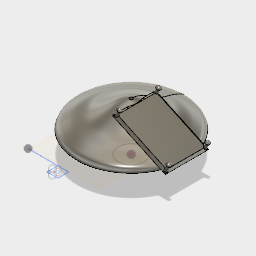
modiTOP v4 (Autodesk Fusion 360 design; units mm, degrees)
Autodesk Fusion 360 part; units mm, degrees
note: some values were not read from the file. Set by a fixed rule: which sketch regions a step uses.
sketch "Sketch1" plane through (0, 0, 0) normal (0, 1, 0) x (1, 0, 0)
  line L0 (-40.284, 39.4847) -> (20.716, 39.4847)
  line L1 (20.716, 39.4847) -> (20.716, -51.0153)
  line L2 (20.716, -51.0153) -> (-40.284, -51.0153)
  line L3 (-40.284, -51.0153) -> (-40.284, 39.4847)
  dimension "d1" = 61
  dimension "d2" = 90.5
  measures "d1" distance of L0.start L0.end
  measures "d2" distance of L0.start L2.end
extrude "Extrude1" add sketch "Sketch1" along normal blind 10 makes body 1
shell "Shell1" thickness 2 outward yes removed faces 1 at (-19.9507, 10, -9.3181) on bodies 1
sketch "Sketch2" plane through (0, 0, 0) normal (0, 1, 0) x (-1, 0, 0)
  line L0 (40.284, 51.0153) -> (-20.716, 51.0153)
  line L1 (-20.716, 51.0153) -> (-20.716, -39.4847)
  line L2 (-20.716, -39.4847) -> (40.284, -39.4847)
  line L3 (40.284, -39.4847) -> (40.284, 51.0153)
  line L4 (40.284, 51.0153) -> (9.784, 51.0153)
  line L5 (9.784, 51.0153) -> (9.784, 5.7653)
  circle A0 centre (9.784, 5.7653) radius 9
  dimension "d6" = 45.25
  dimension "d7" = 18
  measures "d6" distance of L4.end L5.end
  measures "d7" diameter of A0
extrude "Extrude2" cut sketch "Sketch2" against normal blind 3 contours A0 bodies 1
sketch "Sketch3" plane through (0, 10, 0) normal (0, 1, 0) x (-1, 0, 0)
  line L0 (40.284, 51.0153) -> (40.284, -39.4847)
  line L1 (40.284, -39.4847) -> (-20.716, -39.4847)
  line L2 (-20.716, -39.4847) -> (-20.716, 51.0153)
  line L3 (-20.716, 51.0153) -> (40.284, 51.0153)
  line L4 (42.284, 53.0153) -> (-22.716, 53.0153)
  line L5 (-22.716, 53.0153) -> (-22.716, -41.4847)
  line L6 (-22.716, -41.4847) -> (42.284, -41.4847)
  line L7 (42.284, -41.4847) -> (42.284, 53.0153)
  line L8 (42.284, -41.4847) -> (14.784, -41.4847)
  line L9 (14.784, -41.4847) -> (4.784, -41.4847)
  line L10 (4.784, -41.4847) -> (-22.716, -41.4847)
  line L11 (14.784, -41.4847) -> (4.784, -41.4847)
  line L12 (4.784, -41.4847) -> (4.784, -51.4847)
  line L13 (4.784, -51.4847) -> (14.784, -51.4847)
  line L14 (14.784, -51.4847) -> (14.784, -41.4847)
  line L15 (4.784, -51.4847) -> (9.784, -51.4847)
  line L16 (9.784, -51.4847) -> (9.784, -46.4847)
  circle A0 centre (9.784, -46.4847) radius 1.5
  dimension "d10" = 27.5
  dimension "d11" = 10
  dimension "d12" = 27.5
  dimension "d13" = 10
  dimension "d14" = 10
  dimension "d15" = 5
  dimension "d16" = 5
  dimension "d17" = 3
  measures "d10" distance of L6.end L8.end
  measures "d11" distance of L8.end L9.end
  measures "d12" distance of L9.end L5.end
  measures "d13" distance of L8.end L9.end
  measures "d14" distance of L8.end L13.end
  measures "d15" distance of L12.end L15.end
  measures "d16" distance of L15.end L16.end
  measures "d17" diameter of A0
extrude "Extrude3" add sketch "Sketch3" against normal blind 5 contours L6 L9 L11 L12 L13 L14 L15 bodies 1
sketch "Sketch4" plane through (0, 10, 0) normal (0, 1, 0) x (-1, 0, 0)
  circle A0 centre (9.784, -46.4847) radius 1.5
  line L0 (40.284, 51.0153) -> (40.284, -39.4847)
  line L1 (40.284, -39.4847) -> (-20.716, -39.4847)
  line L2 (-20.716, -39.4847) -> (-20.716, 51.0153)
  line L3 (-20.716, 51.0153) -> (40.284, 51.0153)
  line L4 (42.284, 53.0153) -> (-22.716, 53.0153)
  line L5 (-22.716, 53.0153) -> (-22.716, -41.4847)
  line L6 (-22.716, -41.4847) -> (4.784, -41.4847)
  line L7 (4.784, -41.4847) -> (4.784, -51.4847)
  line L8 (4.784, -51.4847) -> (14.784, -51.4847)
  line L9 (14.784, -51.4847) -> (14.784, -41.4847)
  line L10 (14.784, -41.4847) -> (42.284, -41.4847)
  line L11 (42.284, -41.4847) -> (42.284, 53.0153)
  line L12 (42.284, 53.0153) -> (14.784, 53.0153)
  line L13 (14.784, 53.0153) -> (4.784, 53.0153)
  line L14 (4.784, 53.0153) -> (4.784, 63.0153)
  line L15 (4.784, 63.0153) -> (14.784, 63.0153)
  line L16 (14.784, 63.0153) -> (14.784, 53.0153)
  line L17 (14.784, 63.0153) -> (9.784, 63.0153)
  line L18 (14.784, 58.0153) -> (14.784, 63.0153)
  circle A1 centre (9.784, 58.0153) radius 1.5
  dimension "d20" = 27.5
  dimension "d21" = 10
  dimension "d22" = 10
  dimension "d23" = 5
  dimension "d24" = 5
  dimension "d25" = 3
  measures "d20" distance of L4.start L12.end
  measures "d21" distance of L12.end L13.end
  measures "d22" distance of L12.end L15.end
  measures "d23" distance of L15.end L17.end
  measures "d24" distance of L15.end L18.start
  measures "d25" diameter of A1
extrude "Extrude4" add sketch "Sketch4" against normal blind 5 contours L4 L13 L14 L15 L16 L17 L18 bodies 1
sketch "Sketch5" plane through (0, 0, 0) normal (0, 1, 0) x (1, 0, 0)
  circle A0 centre (0, 0) radius 12
  dimension "d28" = 24
  measures "d28" diameter of A0
extrude "Extrude5" add sketch "Sketch5" along normal blind 10 separate body makes body 2
extrude "Extrude6" add 1 faces at (1.8223, 10, -1.3289) along direction (0, 1, 0) blind 10 on bodies 2 bodies 2
shell "Shell2" thickness 2 removed faces 1 at (1.8223, 20, -1.3289) on bodies 2
sketch "Sketch6" plane through (0, 0, 0) normal (1, 0, 0) x (0, 0, -1)
  line L0 (-10, 20) -> (10, 20)
  line L1 (0, 20) -> (0, 45)
  line L2 (0, 20) -> (50, 20)
  spline S0 degree 5 poles (0, 45) (0.3016, 44.9569) (0.8982, 44.8674) (1.7738, 44.7229) (2.9022, 44.5101) (4.2485, 44.21) (5.5325, 43.8749) (6.7585, 43.5032) (7.9341, 43.0921) (9.0709, 42.6377) (10.1838, 42.1352) (11.2892, 41.5803) (12.4029, 40.9706) (13.5381, 40.3065) (14.7037, 39.5927) (15.9035, 38.8381) (17.137, 38.054) (18.3994, 37.2538) (19.6817, 36.4513) (20.9713, 35.6603) (22.2522, 34.8928) (23.5079, 34.1595) (24.7246, 33.4693) (25.8944, 32.8291) (27.018, 32.2438) (28.1088, 31.7161) (29.1922, 31.246) (30.2969, 30.8301) (31.4488, 30.4613) (32.6642, 30.128) (33.941, 29.8131) (35.2609, 29.4959) (36.5968, 29.1563) (37.9194, 28.7782) (39.2032, 28.3529) (40.4343, 27.8835) (41.6132, 27.3855) (42.7472, 26.8789) (43.8449, 26.3817) (44.9104, 25.9032) (45.9361, 25.4363) (46.9006, 24.9552) (47.7763, 24.425) (48.5341, 23.8086) (49.1499, 23.0753) (49.61, 22.207) (49.8482, 21.3973) (49.9528, 20.7243) (49.9897, 20.2463) (50, 20) knots 0 0 0 0 0 0 0.022222 0.044444 0.066667 0.088889 0.111111 0.133333 0.155556 0.177778 0.2 0.222222 0.244444 0.266667 0.288889 0.311111 0.333333 0.355556 0.377778 0.4 0.422222 0.444444 0.466667 0.488889 0.511111 0.533333 0.555556 0.577778 0.6 0.622222 0.644444 0.666667 0.688889 0.711111 0.733333 0.755556 0.777778 0.8 0.822222 0.844444 0.866667 0.888889 0.911111 0.933333 0.955556 0.977778 1 1 1 1 1 1
  point P0 (7.2369, 43.3286)
  point P1 (12.8037, 40.7307)
  point P2 (19.6695, 36.4628)
  point P3 (26.5353, 32.5)
  point P4 (31.9166, 30.3393)
  point P5 (38.7823, 28.4837)
  point P6 (44.5348, 26.0714)
  point P7 (48.4315, 23.8446)
  dimension "d34" = 25
  dimension "d35" = 50
  measures "d34" distance of L1.start L1.end
  measures "d35" distance of L1.start L2.end
revolve "Revolve1" add sketch "Sketch6" angle 360 about axis through (0, 1.75, 0) along (0, 1, 0) bodies 2
sketch "Sketch7" plane through (0, 0, 0) normal (0, -1, 0) x (1, 0, 0)
  circle A0 centre (0, 0) radius 12
  circle A1 centre (0, 0) radius 11
  dimension "d37" = 22
  measures "d37" diameter of A1
extrude "Extrude7" cut sketch "Sketch7" against normal blind 10 contours A1 bodies 2
sketch "Sketch8" plane through (0, 20, 0) normal (0, -1, 0) x (1, 0, 0)
  circle A0 centre (0, 0) radius 10
  circle A1 centre (0, 0) radius 12
  line L0 (0, 0) -> (-6, -10.3923)
  line L1 (0, 0) -> (12, 0) construction
  line L2 (0, 0) -> (6, -10.3923)
  line L3 (0, 0) -> (12, 0) construction
  line L4 (6, -10.3923) -> (6, -13.3923)
  line L5 (6, -13.3923) -> (-6, -13.3923)
  line L6 (-6, -13.3923) -> (-6, -10.3923)
  line L7 (0, 0) -> (-6, 10.3923)
  line L8 (0, 0) -> (12, 0) construction
  line L9 (0, 0) -> (6, 10.3923)
  line L10 (0, 0) -> (12, 0) construction
  line L11 (6, 10.3923) -> (6, 13.3923)
  line L12 (6, 13.3923) -> (-6, 13.3923)
  line L13 (-6, 13.3923) -> (-6, 10.3923)
  dimension "d40" = 24
  dimension "d42" = 120
  dimension "d43" = 60
  dimension "d45" = 3
  dimension "d46" = 120
  dimension "d47" = 60
  dimension "d48" = 3
  measures "d40" diameter of A1
  measures "d42" angle of L0 L1
  measures "d43" angle of L2 L3
  measures "d45" distance of L0.end L5.end
  measures "d46" angle of L7 L8
  measures "d47" angle of L9 L10
  measures "d48" distance of L7.end L12.end
extrude "Extrude8" add sketch "Sketch8" along normal blind 20 contours A1 L11 L12 L13 | A1 L4 L5 L6 bodies 2
sketch "Sketch9" plane through (0, 0, -13.3923) normal (0, 0, -1) x (-1, 0, 0)
  line L0 (6, 20) -> (-6, 20)
  line L1 (-6, 20) -> (-6, 0)
  line L2 (-6, 0) -> (6, 0)
  line L3 (6, 0) -> (6, 20)
  line L4 (6, 0) -> (0, 0)
  line L5 (0, 0) -> (0, 5)
  circle A0 centre (0, 5) radius 1.5
  dimension "d51" = 5
  dimension "d52" = 3
  measures "d51" distance of L4.end L5.end
  measures "d52" diameter of A0
extrude "Extrude9" cut sketch "Sketch9" against normal blind 100 contours A0 bodies 2
extrude "Extrude10" cut sketch "Sketch8" along normal blind 20 contours A1 L11 L12 L13 | A1 L4 L5 L6 bodies 2
sketch "Sketch10" plane through (0, 20, 0) normal (0, -1, 0) x (1, 0, 0)
  circle A0 centre (0, 0) radius 50
  circle A1 centre (0, 0) radius 12
  line L0 (0, 0) -> (0, -20)
  line L1 (0, 0) -> (0, 20)
  line L2 (0, 20) -> (4, 20)
  line L3 (4, 20) -> (4, -20)
  line L4 (4, -20) -> (0, -20)
  line L5 (0, -20) -> (2, -20)
  line L6 (2, -20) -> (2, -18)
  circle A2 centre (2, -18) radius 2
  circle A3 centre (2, -18) radius 1.5
  circle A4 centre (0, 0) radius 1.5
  dimension "d57" = 20
  dimension "d58" = 20
  dimension "d59" = 4
  dimension "d60" = 40
  dimension "d61" = 2
  dimension "d62" = 2
  dimension "d63" = 4
  dimension "d64" = 3
  dimension "d65" = 3
  measures "d57" distance of A0.centre L0.end
  measures "d58" distance of A0.centre L1.end
  measures "d59" distance of L1.end L2.end
  measures "d60" distance of L2.end L3.end
  measures "d61" distance of L0.end L5.end
  measures "d62" distance of L5.end L6.end
  measures "d63" diameter of A2
  measures "d64" diameter of A3
  measures "d65" diameter of A4
extrude "Extrude11" cut sketch "Sketch10" against normal blind 100 contours L0 L1 A4 | L0 L1 A4 bodies 2
sketch "Sketch11" plane through (0, 0, 0) normal (0, 0, 1) x (1, 0, 0)
sketch "Sketch12" plane through (0, 0, 0) normal (0, 1, 0) x (1, 0, 0)
  line L0 (66.4689, 19.1421) -> (120.4689, 19.1421)
  line L1 (120.4689, 19.1421) -> (120.4689, -20.8579)
  line L2 (120.4689, -20.8579) -> (66.4689, -20.8579)
  line L3 (66.4689, -20.8579) -> (66.4689, 19.1421)
  dimension "d68" = 54
  dimension "d69" = 40
  measures "d68" distance of L0.start L0.end
  measures "d69" distance of L0.start L2.end
extrude "Extrude12" add sketch "Sketch12" along normal blind 2 separate body makes body 3
sketch "Sketch13" plane through (0, 2, 0) normal (0, 1, 0) x (-1, 0, 0)
  line L0 (-66.4689, 20.8579) -> (-120.4689, 20.8579)
  line L1 (-120.4689, 20.8579) -> (-120.4689, -19.1421)
  line L2 (-120.4689, -19.1421) -> (-66.4689, -19.1421)
  line L3 (-66.4689, -19.1421) -> (-66.4689, 20.8579)
  line L4 (-66.4689, 20.8579) -> (-70.4689, 20.8579)
  line L5 (-70.4689, 20.8579) -> (-70.4618, -19.1421)
  line L6 (-70.4689, 20.8579) -> (-70.4686, 18.8579)
  line L7 (-70.4686, 18.8579) -> (-68.4686, 18.8582)
  circle A0 centre (-68.4686, 18.8582) radius 1.5
  line L8 (-70.4618, -19.1421) -> (-68.4618, -19.1421)
  line L9 (-68.4618, -19.1421) -> (-68.4618, -17.1421)
  circle A1 centre (-68.4618, -17.1421) radius 1.5
  dimension "d72" = 4
  dimension "d73" = 40
  dimension "d74" = 2
  dimension "d75" = 2
  dimension "d76" = 3
  dimension "d77" = 2
  dimension "d78" = 2
  dimension "d79" = 3
  measures "d72" distance of L0.start L4.end
  measures "d73" distance of L4.end L5.end
  measures "d74" distance of L4.end L6.end
  measures "d75" distance of L6.end L7.end
  measures "d76" diameter of A0
  measures "d77" distance of L5.end L8.end
  measures "d78" distance of L8.end L9.end
  measures "d79" diameter of A1
extrude "Extrude13" add sketch "Sketch13" along normal blind 5 contours A0 | A1 bodies 3
sketch "Sketch14" plane through (0, 7, 0) normal (0, 1, 0) x (-1, 0, 0)
  circle A0 centre (-68.4618, -17.1421) radius 1.5
  circle A1 centre (-68.4618, -17.1421) radius 2
  dimension "d82" = 4
  measures "d82" diameter of A1
extrude "Extrude14" add sketch "Sketch14" along normal blind 2 contours A0 | A1 bodies 3
sketch "Sketch15" plane through (0, 7, 0) normal (0, 1, 0) x (-1, 0, 0)
  circle A0 centre (-68.4686, 18.8582) radius 1.5
  circle A1 centre (-68.4686, 18.8582) radius 2
  dimension "d85" = 4
  measures "d85" diameter of A1
extrude "Extrude15" add sketch "Sketch15" along normal blind 2 contours A0 | A1 bodies 3
sketch "Sketch16" plane through (0, 2, 0) normal (0, 1, 0) x (-1, 0, 0)
  circle A0 centre (-68.4686, 18.8582) radius 1.5
  circle A1 centre (-68.4618, -17.1421) radius 1.5
  line L0 (-66.4689, 20.8579) -> (-120.4689, 20.8579)
  line L1 (-120.4689, 20.8579) -> (-120.4689, -19.1421)
  line L2 (-120.4689, -19.1421) -> (-66.4689, -19.1421)
  line L3 (-66.4689, -19.1421) -> (-66.4689, 20.8579)
  line L4 (-120.4689, 20.8579) -> (-120.4689, 18.8579)
  line L5 (-120.4689, 18.8579) -> (-118.4689, 18.8579)
  circle A2 centre (-118.4689, 18.8579) radius 1.5
  dimension "d88" = 2
  dimension "d89" = 2
  dimension "d90" = 3
  measures "d88" distance of L0.end L4.end
  measures "d89" distance of L4.end L5.end
  measures "d90" diameter of A2
extrude "Extrude16" add sketch "Sketch16" along normal blind 5 contours A2 bodies 3
sketch "Sketch17" plane through (0, 7, 0) normal (0, 1, 0) x (-1, 0, 0)
  circle A0 centre (-118.4689, 18.8579) radius 1.5
  circle A1 centre (-118.4689, 18.8579) radius 2
  dimension "d93" = 4
  measures "d93" diameter of A1
extrude "Extrude17" add sketch "Sketch17" along normal blind 2 contours A0 | A1 bodies 3
sketch "Sketch18" plane through (0, 2, 0) normal (0, 1, 0) x (-1, 0, 0)
  circle A0 centre (-118.4689, 18.8579) radius 1.5
  circle A1 centre (-68.4686, 18.8582) radius 1.5
  circle A2 centre (-68.4618, -17.1421) radius 1.5
  line L0 (-66.4689, 20.8579) -> (-120.4689, 20.8579)
  line L1 (-120.4689, 20.8579) -> (-120.4689, -19.1421)
  line L2 (-120.4689, -19.1421) -> (-66.4689, -19.1421)
  line L3 (-66.4689, -19.1421) -> (-66.4689, 20.8579)
  line L4 (-120.4689, -19.1421) -> (-120.4689, -17.1421)
  line L5 (-120.4689, -17.1421) -> (-118.4689, -17.1421)
  circle A3 centre (-118.4689, -17.1421) radius 1.5
  dimension "d96" = 2
  dimension "d97" = 2
  dimension "d98" = 3
  measures "d96" distance of L1.end L4.end
  measures "d97" distance of L4.end L5.end
  measures "d98" diameter of A3
extrude "Extrude18" add sketch "Sketch18" along normal blind 5 contours A3 bodies 3
sketch "Sketch19" plane through (0, 7, 0) normal (0, 1, 0) x (-1, 0, 0)
  circle A0 centre (-118.4689, -17.1421) radius 1.5
  circle A1 centre (-118.4689, -17.1421) radius 2
  dimension "d101" = 4
  measures "d101" diameter of A1
extrude "Extrude19" add sketch "Sketch19" along normal blind 2 contours A0 | A1 bodies 3
fillet "Fillet1" radius 2 1 edges at (120.3336, 9, 18.1347) on bodies 3
fillet "Fillet2" radius 2 1 edges at (70.3332, 9, 18.135) on bodies 3
fillet "Fillet3" radius 2 1 edges at (70.3264, 9, -17.8653) on bodies 3
fillet "Fillet4" radius 2 1 edges at (120.3336, 9, -17.8653) on bodies 3
move_body "Move1" bodies 3 to x (1, 0, 0) y (0, 1, 0) z (0, 0, 1) at (-64.0221, 41.6652, 0)
move_body "Move2" bodies 3 to x (0.906308, -0.422618, 0) y (0.422618, 0.906308, 0) z (0, 0, 1) at (-16.3637, 6.4591, 0)
combine "Combine1" operation add target body 3 tool bodies 2
chamfer "Chamfer1" distance 2 angle 45 1 edges at (28.7779, 33.5884, -19.1421) on bodies 3
chamfer "Chamfer2" distance 2 angle 45 1 edges at (28.7779, 33.5884, 20.8579) on bodies 3
chamfer "Chamfer3" distance 2 angle 45 1 edges at (4.3076, 44.9991, 0.8579) on bodies 3
chamfer "Chamfer4" distance 2 angle 45 1 edges at (53.2482, 22.1777, 0.8579) on bodies 3
hidden bodies 1
